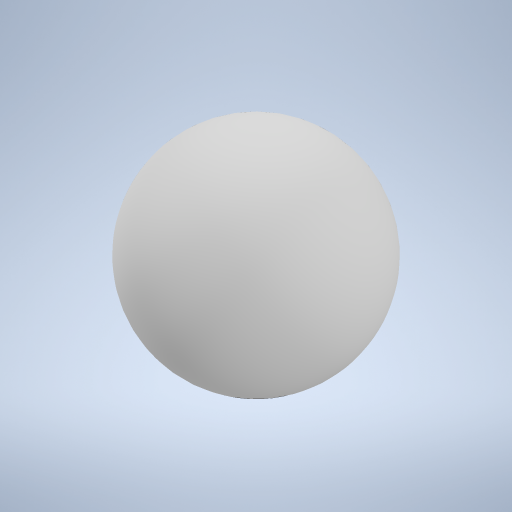
# Autodesk Inventor part: Задание номер 16
Saved by Autodesk Inventor 2023.2 (Build 272271030, 271C)
## iProperties
Created: 2023-09-07
Part Number: Задание номер 16
Material: Типовые
Document SubType Name: Modeling
Designer: User
Density: 1 g/cm^3
Appearance: По умолчанию
Author: User
Autodesk Inventor part; units mm, degrees
ref_plane "YZ Plane" through (0, 0, 0) normal (1, 0, 0) x (0, 1, 0)
ref_plane "XZ Plane" through (0, 0, 0) normal (0, 1, 0) x (-1, 0, 0)
ref_plane "XY Plane" through (0, 0, 0) normal (0, 0, 1) x (1, 0, 0)
sketch "Эскиз1" plane through (0, 0, 0) normal (1, 0, 0) x (0, 1, 0)
  arc A0 (1.6137, 0.113) -> (18.1137, 5.088) centre (9.1137, 5.088) ccw
  line L0 (1.6137, 3.088) -> (5.3137, 3.088)
  line L1 (18.1137, 5.088) -> (5.3137, 5.088)
  line L2 (1.6137, 0.113) -> (1.6137, 3.088)
  line L3 (5.3137, 5.088) -> (5.3137, 3.088)
  point P0 (0, 0)
  dimension "d2" = 3.7
  constraints: 8 end point, 2 point on circle, 2 vertical, 1 centre point
  measures "d2" distance of L0.start L0.end
sketch "Эскиз2" plane through (0, 0, 0) normal (1, 0, 0) x (0, 1, 0)
  point P0 (0, 0)
sketch "Эскиз3" plane through (0, 0, 0) normal (1, 0, 0) x (0, 1, 0)
  point P0 (0, 0)
revolve "Вращение1" add sketch "Эскиз1" angle 360 about axis through (0, 18.1137, 5.088) along (0, -1, 0)
